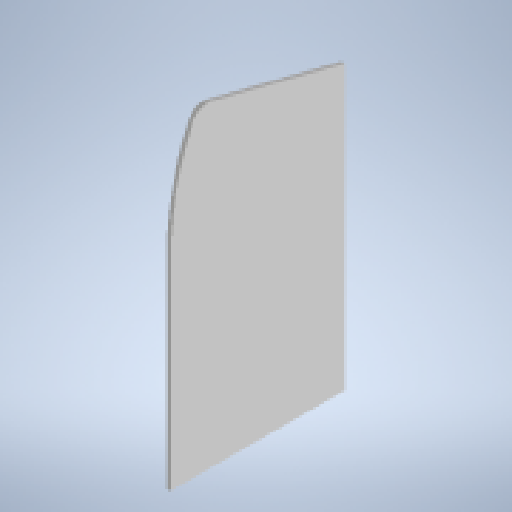
# Autodesk Inventor part: verkleidungBremse
Saved by Autodesk Inventor 2025 (Build 290162010, 162A)
## iProperties
Created: 2025-01-27
Part Number: verkleidungBremse
Material: Generisch
Document SubType Name: Modeling
Designer: Admin
Density: 1 g/cm^3
Appearance: Vorgabe
Author: Admin
Autodesk Inventor part; units mm, degrees
ref_plane "YZ Plane" through (0, 0, 0) normal (1, 0, 0) x (0, 1, 0)
ref_plane "XZ Plane" through (0, 0, 0) normal (0, 1, 0) x (-1, 0, 0)
ref_plane "XY Plane" through (0, 0, 0) normal (0, 0, 1) x (1, 0, 0)
sketch "Skizze1" plane through (0, 0, 0) normal (1, 0, 0) x (0, 1, 0)
  line L0 (19.6888, -8.5435) -> (-13.5827, -0.0073)
  arc A0 (-13.5827, -0.0073) -> (-18.2505, -2.2997) centre (-14.5767, -3.8818) ccw
  arc A1 (-18.2505, -2.2997) -> (-23.6613, -28.5435) centre (42.6888, -28.5435) ccw
  line L1 (-23.6613, -28.5435) -> (-23.6613, -91.5435)
  line L2 (-23.6613, -91.5435) -> (19.6888, -91.5435)
  line L3 (19.6888, -91.5435) -> (19.6888, -8.5435)
  circle A2 centre (42.6888, -28.5435) radius 1.621 projected
  arc A3 (-14.3179, -2.9159) -> (-15.3279, -4.5419) centre (-14.5767, -3.8818) ccw projected
  line L4 (19.6888, -8.5435) -> (19.6888, -44.2151) projected
  line L5 (-23.6613, -28.5435) -> (42.6888, -28.5435) construction
  dimension "d3" = 83
  dimension "d4" = 3
  constraints: 10 end point, 4 point on circle, 3 perpendicular, 2 centre point, 2 coincident, 2 tangent, 1 collinear
  measures "d3" distance of L0.start L2.end
  measures "d4" distance from line of L0 A3.start
extrude "Extrusion1" add sketch "Skizze1" along normal blind 35 contours L3 L2 L1 A1 A0 L0
sketch "Skizze2" plane through (35, 0, 0) normal (1, 0, 0) x (0, 0, -1)
  line L0 (8.5435, 19.6888) -> (9.5759, 19.6888)
  line L1 (9.5759, 19.6888) -> (0.976, -13.8312)
  arc A0 (0.976, -13.8312) -> (2.6952, -17.332) centre (3.8818, -14.5767) ccw
  arc A1 (2.6952, -17.332) -> (28.5435, -22.6613) centre (28.5435, 42.6888) ccw
  line L2 (28.5435, -22.6613) -> (91.5435, -22.6613)
  line L3 (91.5435, 19.6888) -> (8.5435, 19.6888) projected
  line L4 (91.5435, -23.6613) -> (91.5435, 19.6888) projected
  line L5 (28.5435, -23.6613) -> (91.5435, -23.6613) projected
  arc A2 (2.2997, -18.2505) -> (28.5435, -23.6613) centre (28.5435, 42.6888) ccw projected
  arc A3 (0.0073, -13.5827) -> (2.2997, -18.2505) centre (3.8818, -14.5767) ccw projected
  line L6 (8.5435, 19.6888) -> (0.0073, -13.5827) projected
  point P0 (0, 0)
  constraints: 6 end point, 4 point on circle, 3 tangent, 2 centre point, 2 coincident
extrude "Extrusion2" cut sketch "Skizze2" against normal blind 34 contours L3 L4 L2 A1 A0 L1
sketch "Skizze3" plane through (35, 0, 0) normal (1, 0, 0) x (0, 0, -1)
  line L0 (91.5435, 19.6888) -> (8.5435, 19.6888) projected
  line L1 (91.5435, -23.6613) -> (91.5435, 19.6888) projected
  line L2 (28.5435, -23.6613) -> (91.5435, -23.6613) projected
  arc A0 (2.2997, -18.2505) -> (28.5435, -23.6613) centre (28.5435, 42.6888) ccw projected
  arc A1 (0.0073, -13.5827) -> (2.2997, -18.2505) centre (3.8818, -14.5767) ccw projected
  line L3 (8.5435, 19.6888) -> (0.0073, -13.5827) projected
  point P0 (0, 0)
extrude "Extrusion3" add sketch "Skizze3" along normal blind 1
sketch "Skizze6" plane through (1, 0, 0) normal (1, 0, 0) x (0, 0, -1)
  line L0 (9.5759, 19.6888) -> (91.5435, 19.6888) projected
  line L1 (9.5759, 19.6888) -> (19.5759, 19.6888)
  line L2 (19.5759, 19.6888) -> (6.1249, 6.2378)
  line L3 (0.976, -13.8312) -> (9.5759, 19.6888) projected
  point P0 (0, 0)
  dimension "d40" = 10
  dimension "d41" = 45
  constraints: 4 end point, 2 point on line
  measures "d40" distance of L0.start L1.end
  measures "d41" angle of L1 L2
fillet "Rundung1" radius 2 14 edges at (36, -23.6613, -60.0435) (36, -16.34, -0.2914) (36, 3.0531, -4.2754) (36, -22.2945, -15.1456) (0, -23.6613, -60.0435) (0, -16.34, -0.2914) (0, 3.0531, -4.2754) (0, -22.2945, -15.1456) (1, -21.3151, -15.3475) (1, -15.8991, -1.189) (1, 2.9288, -5.2759) (1, -22.6613, -60.0435) (35, -21.3151, -15.3475) (35, -15.8991, -1.189)
sketch "Skizze4" plane through (0, 19.6888, -10.6083) normal (0, 1, 0) x (1, 0, 0)
  line L0 (0, 80.9352) -> (0, 0) projected
  line L1 (0, 80.9352) -> (-7, 80.9352)
  line L2 (-7, 80.9352) -> (-7, 65.9352)
  line L3 (-7, 65.9352) -> (0, 65.9352)
  line L4 (0, 65.9352) -> (0, 80.9352)
  circle A0 centre (-3, 72.5285) radius 0.7835 projected
  line L5 (36, 80.9352) -> (36, 0) projected
  line L6 (36, 80.9352) -> (43, 80.9352)
  line L7 (43, 80.9352) -> (43, 65.9352)
  line L8 (43, 65.9352) -> (36, 65.9352)
  line L9 (36, 65.9352) -> (36, 80.9352)
  circle A1 centre (39, 72.5285) radius 0.7835 projected
  circle A2 centre (-3, 72.5285) radius 1.1
  circle A3 centre (39, 72.5285) radius 1.1
  point P0 (0, -10.6083)
  point P1 (2, 65.9352)
  point P2 (0, -2.0648)
  point P3 (2, -1.0324)
  point P4 (36, 65.9352)
  point P5 (36, 2.9352)
  dimension "d17" = 7
  dimension "d18" = 15
  dimension "d19" = 7
  dimension "d20" = 15
  dimension "d21" = 2.2
  dimension "d22" = 2.2
  constraints: 16 end point, 4 parallel, 2 centre point, 2 coincident, 2 horizontal, 2 perpendicular, 1 other
  measures "d17" distance of L3.end L2.end
  measures "d18" distance of L2.end L1.end
  measures "d19" distance of L7.end L8.end
  measures "d20" distance of L6.end L7.end
  measures "d21" diameter of A2
  measures "d22" diameter of A3
extrude "Extrusion4" add sketch "Skizze4" against normal blind 2 contours L0 L3 L2 L1 | L6 L7 L8 L5
chamfer "Fasen1" distance 1 angle 45 1 edges at (-4.1, 17.6888, -83.1368)
chamfer "Fasen2" distance 1 angle 45 1 edges at (37.9, 17.6888, -83.1368)
extrude "Extrusion7" add sketch "Skizze6" along normal blind 6
sketch "Skizze8" plane through (35, 0, 0) normal (-1, 0, 0) x (0, 0, 1)
  line L0 (-9.5759, 19.6888) -> (-19.5759, 19.6888)
  line L1 (-91.5435, 19.6888) -> (-8.5435, 19.6888) projected
  line L2 (-19.5759, 19.6888) -> (-6.1249, 6.2378)
  line L3 (-0.976, -13.8312) -> (-9.5759, 19.6888) projected
  point P0 (0, 0)
  dimension "d44" = 10
  dimension "d45" = 45
  constraints: 4 end point, 2 point on line
  measures "d44" distance of L0.start L0.end
  measures "d45" angle of L2 L0
extrude "Extrusion8" add sketch "Skizze8" along normal blind 6
